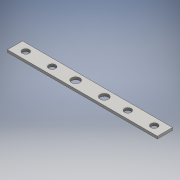
# Autodesk Inventor part: side
Saved by Autodesk Inventor 2016 (Build 200138000, 138)
## iProperties
Created: 2016-09-24
Part Number: side
Material: Generic
Document SubType Name: Modeling
Designer: Kevin G
Density: 1 g/cm^3
Appearance: Default
Author: Kevin G
Autodesk Inventor part; units mm, degrees
ref_plane "YZ Plane" through (0, 0, 0) normal (1, 0, 0) x (0, 1, 0)
ref_plane "XZ Plane" through (0, 0, 0) normal (0, 1, 0) x (-1, 0, 0)
ref_plane "XY Plane" through (0, 0, 0) normal (0, 0, 1) x (1, 0, 0)
sketch "Sketch1" plane through (0, 0, 0) normal (0, 0, 1) x (1, 0, 0)
  line L0 (-99.06, 19.05) -> (469.9, 19.05)
  line L1 (469.9, 19.05) -> (469.9, -38.1)
  line L2 (469.9, -38.1) -> (-99.06, -38.1)
  line L3 (-99.06, -38.1) -> (-99.06, 19.05)
  circle A0 centre (-58.42, -9.525) radius 13
  circle A1 centre (41.716, -9.525) radius 13
  circle A2 centre (131.092, -9.525) radius 16
  circle A3 centre (429.26, -9.525) radius 13
  circle A4 centre (329.124, -9.525) radius 13
  circle A5 centre (239.748, -9.525) radius 16
  point P0 (0, 0)
  dimension "d4" = 26
  dimension "d6" = 26
  dimension "d8" = 32
  dimension "d10" = 26
  dimension "d12" = 26
  dimension "d14" = 32
  dimension "d16" = 568.96
  dimension "d17" = 57.15
  dimension "d18" = 40.64
  dimension "d19" = 140.776
  dimension "d20" = 230.152
  dimension "d21" = 230.152
  dimension "d22" = 40.64
  dimension "d23" = 140.776
  constraints: 8 end point, 6 centre point, 2 parallel, 1 horizontal, 1 perpendicular
  measures "d4" diameter of A0
  measures "d6" diameter of A1
  measures "d8" diameter of A2
  measures "d10" diameter of A3
  measures "d12" diameter of A4
  measures "d14" diameter of A5
  measures "d16" distance between parallel lines of L1 L3
  measures "d17" distance between parallel lines of L2 L0
  measures "d18" distance from line of A0.centre L3
  measures "d19" distance from line of A1.centre L3
  measures "d20" distance from line of A2.centre L3
  measures "d21" distance from line of A5.centre L1
  measures "d22" distance from line of A3.centre L1
  measures "d23" distance from line of A4.centre L1
extrude "Extrusion1" add sketch "Sketch1" along normal blind 9.525
body "Solid1"
